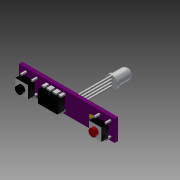
# Autodesk Inventor part: LED Indicator
Saved by Autodesk Inventor 2014 (Build 180170000, 170)
## iProperties
Created: 2014-03-02
Part Number: LED Indicator
Material: Generic
Document SubType Name: Modeling
Designer: Alex
Density: 1 g/cm^3
Appearance: Silver
Author: Alex
Autodesk Inventor part; units mm, degrees
sketch "Sketch4" plane through (0, 0, 0) normal (0, 0, 1) x (1, 0, 0)
  line L0 (0, 0) -> (46.736, 0)
  line L1 (46.736, 0) -> (46.736, 10.16)
  line L2 (46.736, 10.16) -> (0, 10.16)
  line L3 (0, 10.16) -> (0, 0)
  dimension "d6" = 46.736
  dimension "d7" = 10.16
  constraints: 8 end point, 2 parallel, 1 horizontal, 1 perpendicular
  measures "d6" distance of L0.start L0.end
  measures "d7" distance of L2.end L0.start
extrude "Extrusion4" add sketch "Sketch4" along normal blind 1.651
ref_plane "Work Plane2" through (0, 0, 3.175) normal (0, 0, 1) x (1, 0, 0)
sketch "Sketch6" plane through (0, 0, 3.175) normal (0, 0, 1) x (1, 0, 0)
  line L0 (38.989, 2.032) -> (45.085, 2.032)
  line L1 (45.085, 2.032) -> (45.085, 8.128)
  line L2 (45.085, 8.128) -> (38.989, 8.128)
  line L3 (38.989, 8.128) -> (38.989, 2.032)
  line L4 (0, 0) -> (46.736, 0) projected
  line L5 (46.736, 0) -> (46.736, 10.16) projected
  line L6 (46.736, 10.16) -> (0, 10.16) projected
  line L7 (0, 10.16) -> (0, 0) projected
  dimension "d17" = 6.096
  dimension "d18" = 6.096
  dimension "d22" = 2.032
  dimension "d23" = 2.032
  dimension "d24" = 1.651
  constraints: 8 end point, 2 parallel, 1 horizontal, 1 perpendicular
  measures "d17" distance of L1.end L2.end
  measures "d18" distance of L0.end L1.end
  measures "d22" distance between parallel lines of L6 L2
  measures "d23" distance between parallel lines of L4 L0
  measures "d24" distance between parallel lines of L5 L1
extrude "Extrusion5" add sketch "Sketch6" along normal blind 3.302 contours L3 L2 L1 L0
sketch "Sketch7" plane through (0, 0, 6.477) normal (0, 0, 1) x (1, 0, 0)
  line L0 (38.989, 2.032) -> (45.085, 2.032) projected
  line L1 (38.989, 8.128) -> (38.989, 2.032) projected
  circle A0 centre (42.037, 5.08) radius 1.778
  point P0 (45.085, 8.128)
  point P1 (0, 0)
  dimension "d27" = 3.556
  dimension "d28" = 3.048
  dimension "d29" = 6.096
  dimension "d30" = 6.096
  dimension "d31" = 3.048
  constraints: 1 centre point
  measures "d27" diameter of A0
  measures "d28" distance from line of L1 A0.centre
  measures "d29" distance of point (45.085, 8.128) L1.start
  measures "d30" distance of L0.end point (45.085, 8.128)
  measures "d31" distance from line of L0 A0.centre
extrude "Extrusion6" add sketch "Sketch7" along normal blind 1.524
hole "Hole1" at (35.56, 5.08, 1.651) direction (0, 0, -1) diameter 2.921 end through all
sketch "Sketch8" plane through (0, 0, 3.175) normal (0, 0, 1) x (1, 0, 0)
  circle A0 centre (35.56, 5.08) radius 1.4605 projected
  line L0 (0, 0) -> (46.736, 0) projected
  line L1 (46.736, 0) -> (46.736, 10.16) projected
  line L2 (46.736, 10.16) -> (0, 10.16) projected
  line L3 (0, 10.16) -> (0, 0) projected
  line L4 (3.048, 2.032) -> (9.144, 2.032)
  line L5 (9.144, 2.032) -> (9.144, 8.128)
  line L6 (9.144, 8.128) -> (3.048, 8.128)
  line L7 (3.048, 8.128) -> (3.048, 2.032)
  dimension "d43" = 3.048
  dimension "d44" = 2.032
  dimension "d45" = 6.096
  dimension "d46" = 6.096
  constraints: 8 end point, 2 parallel, 1 horizontal, 1 perpendicular
  measures "d43" distance between parallel lines of L3 L7
  measures "d44" distance between parallel lines of L2 L6
  measures "d45" distance of L6.end L4.start
  measures "d46" distance of L5.end L6.end
extrude "Extrusion7" add sketch "Sketch8" along normal blind 3.302 contours L7 L6 L5 L4
sketch "Sketch9" plane through (0, 0, 6.477) normal (0, 0, 1) x (1, 0, 0)
  line L0 (3.048, 2.032) -> (9.144, 2.032) projected
  line L1 (9.144, 2.032) -> (9.144, 8.128) projected
  circle A0 centre (6.096, 5.08) radius 1.778
  point P0 (0, 0)
  dimension "d49" = 3.048
  dimension "d50" = 3.048
  dimension "d51" = 3.556
  constraints: 1 centre point
  measures "d49" distance from line of L1 A0.centre
  measures "d50" distance from line of L0 A0.centre
  measures "d51" diameter of A0
extrude "Extrusion8" add sketch "Sketch9" along normal blind 1.524
ref_plane "Work Plane3" through (0, 0, 2.159) normal (0, 0, 1) x (1, 0, 0)
sketch "Sketch11" plane through (0, 0, 2.159) normal (0, 0, 1) x (1, 0, 0)
  circle A0 centre (35.56, 5.08) radius 1.4605 projected
  line L0 (0, 0) -> (46.736, 0) projected
  line L1 (46.736, 0) -> (46.736, 10.16) projected
  line L2 (46.736, 10.16) -> (0, 10.16) projected
  line L3 (0, 10.16) -> (0, 0) projected
  circle A1 centre (6.096, 5.08) radius 1.778 projected
  line L4 (3.048, 2.032) -> (9.144, 2.032) projected
  line L5 (9.144, 2.032) -> (9.144, 8.128) projected
  line L6 (9.144, 8.128) -> (3.048, 8.128) projected
  line L7 (3.048, 8.128) -> (3.048, 2.032) projected
  line L8 (13.335, 2.032) -> (22.733, 2.032)
  line L9 (22.733, 2.032) -> (22.733, 8.128)
  line L10 (22.733, 8.128) -> (13.335, 8.128)
  line L11 (13.335, 8.128) -> (13.335, 2.032)
  dimension "d67" = 4.191
  dimension "d68" = 6.096
  dimension "d69" = 2.032
  dimension "d70" = 9.398
  constraints: 8 end point, 2 parallel, 1 horizontal, 1 perpendicular
  measures "d67" distance between parallel lines of L11 L5
  measures "d68" distance of L10.end L8.start
  measures "d69" distance between parallel lines of L2 L10
  measures "d70" distance between parallel lines of L9 L11
extrude "Extrusion10" add sketch "Sketch11" along normal blind 3.556 contours L11 L10 L9 L8
ref_plane "Work Plane4" through (0, 0, -18.415) normal (0, 0, -1) x (-1, 0, 0)
sketch "Sketch12" plane through (0, 0, -18.415) normal (0, 0, -1) x (-1, 0, 0)
  circle A0 centre (-35.56, 5.08) radius 1.4605 projected
  line L0 (0, 0) -> (-46.736, 0) projected
  line L1 (0, 10.16) -> (0, 0) projected
  line L2 (-46.736, 10.16) -> (0, 10.16) projected
  line L3 (-46.736, 0) -> (-46.736, 10.16) projected
  circle A1 centre (-25.146, 5.08) radius 2.54
  dimension "d74" = 5.08
  dimension "d75" = 21.59
  dimension "d76" = 5.08
  constraints: 1 centre point
  measures "d74" diameter of A1
  measures "d75" distance from line of L3 A1.centre
  measures "d76" distance from line of L2 A1.centre
extrude "Extrusion11" add sketch "Sketch12" along normal blind 8.89 contours A1
sketch "Sketch13" plane through (0, 0, -18.415) normal (0, 0, -1) x (-1, 0, 0)
  circle A0 centre (-25.146, 5.08) radius 2.54 projected
  circle A1 centre (-25.146, 5.08) radius 2.9845
  circle A2 centre (-25.146, 5.08) radius 2.54
  line L0 (-23.579, 2.54) -> (-26.713, 2.54)
  point P0 (0, 0)
  dimension "d79" = 5.969
  constraints: 2 centre point, 2 coincident, 2 end point, 2 point on circle, 1 concentric, 1 horizontal, 1 tangent
  measures "d79" diameter of A1
extrude "Extrusion13" add sketch "Sketch13" along normal blind 1.016 contours L0 A1 picked at (-22.3393, 5.321)
fillet "Fillet1" radius 2.54 1 edges at (27.686, 5.08, -27.305)
sketch "Sketch14" plane through (0, 0, -18.415) normal (0, 0, 1) x (1, 0, 0)
  arc A0 (26.713, 2.54) -> (23.579, 2.54) centre (25.146, 5.08) ccw projected
  line L0 (24.8285, 7.8105) -> (25.4635, 7.8105)
  line L1 (25.4635, 7.8105) -> (25.4635, 7.1755)
  line L2 (25.4635, 7.1755) -> (24.8285, 7.1755)
  line L3 (24.8285, 7.1755) -> (24.8285, 7.8105)
  line L4 (24.8285, 6.4135) -> (25.4635, 6.4135)
  line L5 (25.4635, 6.4135) -> (25.4635, 5.7785)
  line L6 (25.4635, 5.7785) -> (24.8285, 5.7785)
  line L7 (24.8285, 5.7785) -> (24.8285, 6.4135)
  line L8 (24.8285, 5.0165) -> (25.4635, 5.0165)
  line L9 (25.4635, 5.0165) -> (25.4635, 4.3815)
  line L10 (25.4635, 4.3815) -> (24.8285, 4.3815)
  line L11 (24.8285, 4.3815) -> (24.8285, 5.0165)
  line L12 (24.8285, 3.6195) -> (25.4635, 3.6195)
  line L13 (25.4635, 3.6195) -> (25.4635, 2.9845)
  line L14 (25.4635, 2.9845) -> (24.8285, 2.9845)
  line L15 (24.8285, 2.9845) -> (24.8285, 3.6195)
  point P0 (0, 0)
  point P1 (24.8285, 3.302)
  point P2 (24.8285, 4.699)
  point P3 (24.8285, 6.096)
  point P4 (24.8285, 7.493)
  point P5 (25.146, 7.1755)
  point P6 (25.146, 5.7785)
  dimension "d85" = 0.635
  dimension "d88" = 0.3175
  dimension "d89" = 0.254
  dimension "d90" = 0.762
  dimension "d91" = 0.762
  dimension "d92" = 0.762
  constraints: 32 end point, 8 parallel, 7 equal length, 6 midpoint, 4 horizontal, 4 perpendicular, 4 vertical alignment
  measures "d85" distance of L12.end L13.end
  measures "d88" distance from line of A0.centre L15
  measures "d89" distance edge to line of A0 L0
  measures "d90" distance between parallel lines of L2 L4
  measures "d91" distance between parallel lines of L6 L8
  measures "d92" distance between parallel lines of L10 L12
extrude "Extrusion14" add sketch "Sketch14" along normal up to next
sketch "Sketch16" plane through (0, 0, 1.651) normal (0, 0, 1) x (1, 0, 0)
  circle A0 centre (6.096, 5.08) radius 1.778 projected
  line L0 (3.048, 2.032) -> (9.144, 2.032) projected
  line L1 (9.144, 2.032) -> (9.144, 8.128) projected
  line L2 (9.144, 8.128) -> (3.048, 8.128) projected
  line L3 (3.048, 8.128) -> (3.048, 2.032) projected
  line L4 (13.335, 2.032) -> (22.733, 2.032) projected
  line L5 (22.733, 2.032) -> (22.733, 8.128) projected
  line L6 (22.733, 8.128) -> (13.335, 8.128) projected
  line L7 (13.335, 8.128) -> (13.335, 2.032) projected
  circle A1 centre (42.037, 5.08) radius 1.778 projected
  line L8 (38.989, 2.032) -> (45.085, 2.032) projected
  line L9 (45.085, 2.032) -> (45.085, 8.128) projected
  line L10 (45.085, 8.128) -> (38.989, 8.128) projected
  line L11 (38.989, 8.128) -> (38.989, 2.032) projected
  line L12 (3.048, 8.128) -> (3.81, 8.128)
  line L13 (3.81, 8.128) -> (3.81, 8.89)
  line L14 (3.81, 8.89) -> (3.048, 8.89)
  line L15 (3.048, 8.89) -> (3.048, 8.128)
  line L16 (9.144, 8.128) -> (8.382, 8.128)
  line L17 (8.382, 8.128) -> (8.382, 8.89)
  line L18 (8.382, 8.89) -> (9.144, 8.89)
  line L19 (9.144, 8.89) -> (9.144, 8.128)
  line L20 (3.048, 2.032) -> (3.81, 2.032)
  line L21 (3.81, 2.032) -> (3.81, 1.27)
  line L22 (3.81, 1.27) -> (3.048, 1.27)
  line L23 (3.048, 1.27) -> (3.048, 2.032)
  line L24 (9.144, 2.032) -> (8.382, 2.032)
  line L25 (8.382, 2.032) -> (8.382, 1.27)
  line L26 (8.382, 1.27) -> (9.144, 1.27)
  line L27 (9.144, 1.27) -> (9.144, 2.032)
  line L28 (38.989, 2.032) -> (39.751, 2.032)
  line L29 (39.751, 2.032) -> (39.751, 1.27)
  line L30 (39.751, 1.27) -> (38.989, 1.27)
  line L31 (38.989, 1.27) -> (38.989, 2.032)
  line L32 (45.085, 2.032) -> (44.323, 2.032)
  line L33 (44.323, 2.032) -> (44.323, 1.27)
  line L34 (44.323, 1.27) -> (45.085, 1.27)
  line L35 (45.085, 1.27) -> (45.085, 2.032)
  line L36 (45.085, 8.128) -> (44.323, 8.128)
  line L37 (44.323, 8.128) -> (44.323, 8.89)
  line L38 (44.323, 8.89) -> (45.085, 8.89)
  line L39 (45.085, 8.89) -> (45.085, 8.128)
  line L40 (38.989, 8.128) -> (39.751, 8.128)
  line L41 (39.751, 8.128) -> (39.751, 8.89)
  line L42 (39.751, 8.89) -> (38.989, 8.89)
  line L43 (38.989, 8.89) -> (38.989, 8.128)
  line L44 (13.335, 8.128) -> (14.605, 8.128)
  line L45 (14.605, 8.128) -> (14.605, 8.89)
  line L46 (14.605, 8.89) -> (13.335, 8.89)
  line L47 (13.335, 8.89) -> (13.335, 8.128)
  line L48 (22.733, 8.128) -> (21.463, 8.128)
  line L49 (21.463, 8.128) -> (21.463, 8.89)
  line L50 (21.463, 8.89) -> (22.733, 8.89)
  line L51 (22.733, 8.89) -> (22.733, 8.128)
  line L52 (15.621, 8.128) -> (17.526, 8.128)
  line L53 (17.526, 8.128) -> (17.526, 8.89)
  line L54 (17.526, 8.89) -> (15.621, 8.89)
  line L55 (15.621, 8.89) -> (15.621, 8.128)
  line L56 (18.542, 8.128) -> (20.447, 8.128)
  line L57 (20.447, 8.128) -> (20.447, 8.89)
  line L58 (20.447, 8.89) -> (18.542, 8.89)
  line L59 (18.542, 8.89) -> (18.542, 8.128)
  line L60 (13.335, 2.032) -> (14.605, 2.032)
  line L61 (14.605, 2.032) -> (14.605, 1.27)
  line L62 (14.605, 1.27) -> (13.335, 1.27)
  line L63 (13.335, 1.27) -> (13.335, 2.032)
  line L64 (15.621, 2.032) -> (17.526, 2.032)
  line L65 (17.526, 2.032) -> (17.526, 1.27)
  line L66 (17.526, 1.27) -> (15.621, 1.27)
  line L67 (15.621, 1.27) -> (15.621, 2.032)
  line L68 (18.542, 2.032) -> (20.447, 2.032)
  line L69 (20.447, 2.032) -> (20.447, 1.27)
  line L70 (20.447, 1.27) -> (18.542, 1.27)
  line L71 (18.542, 1.27) -> (18.542, 2.032)
  line L72 (22.733, 2.032) -> (21.463, 2.032)
  line L73 (21.463, 2.032) -> (21.463, 1.27)
  line L74 (21.463, 1.27) -> (22.733, 1.27)
  line L75 (22.733, 1.27) -> (22.733, 2.032)
  point P0 (15.621, 1.651)
  point P1 (15.621, 8.509)
  point P2 (18.542, 1.651)
  point P3 (18.542, 8.509)
  dimension "d95" = 0.762
  dimension "d96" = 1.27
  dimension "d97" = 1.905
  dimension "d98" = 1.016
  dimension "d99" = 1.016
  dimension "d100" = 1.016
  constraints: 128 end point, 32 parallel, 29 equal length, 16 horizontal, 16 perpendicular, 4 midpoint, 4 point on line, 2 vertical alignment
  measures "d95" distance of L13.end L14.end
  measures "d96" distance of L45.end L46.end
  measures "d97" distance of L53.end L54.end
  measures "d98" distance between parallel lines of L55 L45
  measures "d99" distance between parallel lines of L59 L53
  measures "d100" distance between parallel lines of L49 L57
extrude "Extrusion15" add sketch "Sketch16" along normal blind 2.54 contours L0 L21 L22 L23 | L15 L14 L13 L2 | L0 L27 L26 L25 | L17 L18 L19 L2 | L8 L29 L30 L31 | L43 L42 L41 L10 | L8 L35 L34 L33 | L37 L38 L39 L10
sketch "Sketch17" plane through (45.085, 2.032, 6.477) normal (1, 0, 0) x (0, 0, -1)
  line L0 (2.286, -0.762) -> (2.286, 0) projected
  line L1 (4.826, -0.762) -> (2.286, -0.762) projected
  line L2 (2.286, 6.096) -> (4.826, 6.096)
  line L3 (4.826, 6.096) -> (4.826, 6.858)
  line L4 (4.826, 6.858) -> (2.286, 6.858)
  line L5 (2.286, 6.858) -> (2.286, 6.096)
  line L6 (2.286, 0) -> (4.826, 0)
  line L7 (4.826, 0) -> (4.826, -0.762)
  line L8 (4.826, -0.762) -> (2.286, -0.762)
  line L9 (2.286, -0.762) -> (2.286, 0)
  point P0 (6.477, -2.032)
  constraints: 16 end point, 4 parallel, 2 horizontal, 2 perpendicular
extrude "Extrusion16" cut sketch "Sketch17" against normal blind 0.0254
sketch "Sketch18" plane through (38.989, 2.032, 6.477) normal (-1, 0, 0) x (0, 0, 1)
  line L0 (-2.286, 6.858) -> (-2.286, 6.096) projected
  line L1 (-4.826, 6.858) -> (-2.286, 6.858) projected
  line L2 (-2.286, 6.096) -> (-4.826, 6.096)
  line L3 (-4.826, 6.096) -> (-4.826, 6.858)
  line L4 (-4.826, 6.858) -> (-2.286, 6.858)
  line L5 (-2.286, 6.858) -> (-2.286, 6.096)
  line L6 (-2.286, -0.762) -> (-4.826, -0.762)
  line L7 (-4.826, -0.762) -> (-4.826, 0)
  line L8 (-4.826, 0) -> (-2.286, 0)
  line L9 (-2.286, 0) -> (-2.286, -0.762)
  point P0 (-6.477, -2.032)
  constraints: 16 end point, 4 parallel, 2 horizontal, 2 perpendicular
extrude "Extrusion17" cut sketch "Sketch18" against normal blind 0.0254
sketch "Sketch19" plane through (9.144, 2.032, 6.477) normal (1, 0, 0) x (0, 0, -1)
  line L0 (2.286, -0.762) -> (2.286, 0) projected
  line L1 (4.826, -0.762) -> (2.286, -0.762) projected
  line L2 (4.826, 6.096) -> (2.286, 6.096)
  line L3 (2.286, 6.096) -> (2.286, 6.858)
  line L4 (2.286, 6.858) -> (4.826, 6.858)
  line L5 (4.826, 6.858) -> (4.826, 6.096)
  line L6 (4.826, -0.762) -> (2.286, -0.762)
  line L7 (2.286, -0.762) -> (2.286, 0)
  line L8 (2.286, 0) -> (4.826, 0)
  line L9 (4.826, 0) -> (4.826, -0.762)
  point P0 (6.477, -2.032)
  constraints: 16 end point, 4 parallel, 2 horizontal, 2 perpendicular
extrude "Extrusion18" cut sketch "Sketch19" against normal blind 0.0254
sketch "Sketch20" plane through (3.048, 2.032, 6.477) normal (-1, 0, 0) x (0, 0, 1)
  line L0 (-4.826, 6.858) -> (-2.286, 6.858) projected
  line L1 (-4.826, 6.096) -> (-4.826, 6.858) projected
  line L2 (-4.826, 6.096) -> (-2.286, 6.096)
  line L3 (-2.286, 6.096) -> (-2.286, 6.858)
  line L4 (-2.286, 6.858) -> (-4.826, 6.858)
  line L5 (-4.826, 6.858) -> (-4.826, 6.096)
  line L6 (-2.286, 0) -> (-4.826, 0)
  line L7 (-4.826, 0) -> (-4.826, -0.762)
  line L8 (-4.826, -0.762) -> (-2.286, -0.762)
  line L9 (-2.286, -0.762) -> (-2.286, 0)
  point P0 (-6.477, -2.032)
  constraints: 16 end point, 4 parallel, 2 horizontal, 2 perpendicular
extrude "Extrusion19" cut sketch "Sketch20" against normal blind 0.0254
sketch "Sketch21" plane through (0, 0, 1.651) normal (0, 0, 1) x (1, 0, 0)
  line L0 (46.736, 0) -> (46.736, 10.16) projected
  line L1 (46.736, 10.16) -> (0, 10.16) projected
  line L2 (0, 10.16) -> (0, 0) projected
  line L3 (3.048, 2.032) -> (9.144, 2.032)
  line L4 (9.144, 2.032) -> (9.144, 8.128)
  line L5 (9.144, 8.128) -> (3.048, 8.128)
  line L6 (3.048, 8.128) -> (3.048, 2.032)
  line L7 (13.335, 2.032) -> (22.733, 2.032)
  line L8 (22.733, 2.032) -> (22.733, 8.128)
  line L9 (22.733, 8.128) -> (13.335, 8.128)
  line L10 (13.335, 8.128) -> (13.335, 2.032)
  line L11 (3.048, 8.128) -> (3.81, 8.128)
  line L12 (3.81, 8.128) -> (3.81, 8.89)
  line L13 (3.81, 8.89) -> (3.048, 8.89)
  line L14 (3.048, 8.89) -> (3.048, 8.128)
  line L15 (9.144, 8.128) -> (8.382, 8.128)
  line L16 (8.382, 8.128) -> (8.382, 8.89)
  line L17 (8.382, 8.89) -> (9.144, 8.89)
  line L18 (9.144, 8.89) -> (9.144, 8.128)
  line L19 (3.048, 2.032) -> (3.81, 2.032)
  line L20 (3.81, 2.032) -> (3.81, 1.27)
  line L21 (3.81, 1.27) -> (3.048, 1.27)
  line L22 (3.048, 1.27) -> (3.048, 2.032)
  line L23 (9.144, 2.032) -> (8.382, 2.032)
  line L24 (8.382, 2.032) -> (8.382, 1.27)
  line L25 (8.382, 1.27) -> (9.144, 1.27)
  line L26 (9.144, 1.27) -> (9.144, 2.032)
  line L27 (13.335, 8.128) -> (14.605, 8.128)
  line L28 (14.605, 8.128) -> (14.605, 8.89)
  line L29 (14.605, 8.89) -> (13.335, 8.89)
  line L30 (13.335, 8.89) -> (13.335, 8.128)
  line L31 (22.733, 8.128) -> (21.463, 8.128)
  line L32 (21.463, 8.128) -> (21.463, 8.89)
  line L33 (21.463, 8.89) -> (22.733, 8.89)
  line L34 (22.733, 8.89) -> (22.733, 8.128)
  line L35 (15.621, 8.128) -> (17.526, 8.128)
  line L36 (17.526, 8.128) -> (17.526, 8.89)
  line L37 (17.526, 8.89) -> (15.621, 8.89)
  line L38 (15.621, 8.89) -> (15.621, 8.128)
  line L39 (18.542, 8.128) -> (20.447, 8.128)
  line L40 (20.447, 8.128) -> (20.447, 8.89)
  line L41 (20.447, 8.89) -> (18.542, 8.89)
  line L42 (18.542, 8.89) -> (18.542, 8.128)
  line L43 (13.335, 2.032) -> (14.605, 2.032)
  line L44 (14.605, 2.032) -> (14.605, 1.27)
  line L45 (14.605, 1.27) -> (13.335, 1.27)
  line L46 (13.335, 1.27) -> (13.335, 2.032)
  line L47 (15.621, 2.032) -> (17.526, 2.032)
  line L48 (17.526, 2.032) -> (17.526, 1.27)
  line L49 (17.526, 1.27) -> (15.621, 1.27)
  line L50 (15.621, 1.27) -> (15.621, 2.032)
  line L51 (18.542, 2.032) -> (20.447, 2.032)
  line L52 (20.447, 2.032) -> (20.447, 1.27)
  line L53 (20.447, 1.27) -> (18.542, 1.27)
  line L54 (18.542, 1.27) -> (18.542, 2.032)
  line L55 (22.733, 2.032) -> (21.463, 2.032)
  line L56 (21.463, 2.032) -> (21.463, 1.27)
  line L57 (21.463, 1.27) -> (22.733, 1.27)
  line L58 (22.733, 1.27) -> (22.733, 2.032)
  point P0 (15.621, 1.651)
  point P1 (15.621, 8.509)
  point P2 (18.542, 1.651)
  point P3 (18.542, 8.509)
  dimension "d111" = 0.762
  dimension "d112" = 1.27
  dimension "d113" = 1.905
  dimension "d114" = 1.016
  dimension "d115" = 1.016
  dimension "d116" = 1.016
  dimension "d117" = 2.032
  dimension "d118" = 3.048
  dimension "d119" = 6.096
  dimension "d120" = 4.191
  dimension "d121" = 9.144
  dimension "d122" = 2.032
  dimension "d123" = 6.096
  dimension "d124" = 24.003
  constraints: 112 end point, 24 parallel, 21 equal length, 12 horizontal, 12 perpendicular, 4 midpoint, 4 point on line, 2 vertical alignment
  measures "d111" distance of L12.end L13.end
  measures "d112" distance of L28.end L29.end
  measures "d113" distance of L36.end L37.end
  measures "d114" distance between parallel lines of L38 L28
  measures "d115" distance between parallel lines of L42 L36
  measures "d116" distance between parallel lines of L32 L40
  measures "d117" distance between parallel lines of L1 L5
  measures "d118" distance between parallel lines of L2 L6
  measures "d119" distance between parallel lines of L5 L3
  measures "d120" distance between parallel lines of L10 L4
  measures "d121" distance between parallel lines of L2 L4
  measures "d122" distance between parallel lines of L1 L9
  measures "d123" distance between parallel lines of L9 L7
  measures "d124" distance between parallel lines of L0 L8
extrude "Extrusion20" add sketch "Sketch21" along normal blind 2.286 contours L7 L44 L45 L46 | L30 L29 L28 L9 | L7 L48 L49 L50 | L38 L37 L36 L9 | L7 L52 L53 L54 | L42 L41 L40 L9 | L7 L58 L57 L56 | L32 L33 L34 L9
sketch "Sketch22" plane through (22.733, 2.032, 5.715) normal (1, 0, 0) x (0, 0, -1)
  line L0 (1.778, -0.762) -> (1.778, 0) projected
  line L1 (4.064, -0.762) -> (1.778, -0.762) projected
  line L2 (1.778, 6.096) -> (4.064, 6.096)
  line L3 (4.064, 6.096) -> (4.064, 6.858)
  line L4 (4.064, 6.858) -> (1.778, 6.858)
  line L5 (1.778, 6.858) -> (1.778, 6.096)
  line L6 (4.064, -0.762) -> (1.778, -0.762)
  line L7 (1.778, -0.762) -> (1.778, 0)
  line L8 (1.778, 0) -> (4.064, 0)
  line L9 (4.064, 0) -> (4.064, -0.762)
  point P0 (5.715, -2.032)
  constraints: 16 end point, 4 parallel, 2 horizontal, 2 perpendicular
extrude "Extrusion21" cut sketch "Sketch22" against normal blind 0.0254
sketch "Sketch23" plane through (13.335, 2.032, 5.715) normal (-1, 0, 0) x (0, 0, 1)
  line L0 (-1.778, 6.858) -> (-1.778, 6.096) projected
  line L1 (-4.064, 6.858) -> (-1.778, 6.858) projected
  line L2 (-1.778, 6.096) -> (-4.064, 6.096)
  line L3 (-4.064, 6.096) -> (-4.064, 6.858)
  line L4 (-4.064, 6.858) -> (-1.778, 6.858)
  line L5 (-1.778, 6.858) -> (-1.778, 6.096)
  line L6 (-4.064, -0.762) -> (-1.778, -0.762)
  line L7 (-1.778, -0.762) -> (-1.778, 0)
  line L8 (-1.778, 0) -> (-4.064, 0)
  line L9 (-4.064, 0) -> (-4.064, -0.762)
  point P0 (-5.715, -2.032)
  constraints: 16 end point, 4 parallel, 2 horizontal, 2 perpendicular
extrude "Extrusion22" add sketch "Sketch23" along normal blind 0.0254
equation "\"d22\" = d23"
equation "\"d28\" = 0.5 * d29"
equation "\"d31\" = 0.5 * d30"
body "Solid2"
